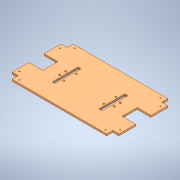
# Autodesk Inventor part: base
Saved by Autodesk Inventor 2020 (Build 240168000, 168)
## iProperties
Part Number: base
Material: Bois (cerisier)
Document SubType Name: Modeling
Designer: ElsaT
Density: 0.63 g/cm^3
Appearance: Cerisier - Faible lustre naturel
Author: ElsaT
Autodesk Inventor part; units mm, degrees
ref_plane "YZ Plane" through (0, 0, 0) normal (1, 0, 0) x (0, 1, 0)
ref_plane "XZ Plane" through (0, 0, 0) normal (0, 1, 0) x (-1, 0, 0)
ref_plane "XY Plane" through (0, 0, 0) normal (0, 0, 1) x (1, 0, 0)
sketch "Esquisse1" plane through (0, 0, 0) normal (0, 0, 1) x (1, 0, 0)
  line L0 (-155, -100) -> (155, -100)
  line L1 (175, -80) -> (175, 80)
  line L2 (155, 100) -> (-155, 100)
  line L3 (-175, 80) -> (-175, -80)
  line L4 (-175, -100) -> (175, 100) construction
  line L5 (175, -100) -> (-175, 100) construction
  line L6 (-155, 100) -> (-155, 80)
  line L7 (-155, 80) -> (-175, 80)
  line L8 (155, 100) -> (155, 80)
  line L9 (155, 80) -> (175, 80)
  line L10 (155, -100) -> (155, -80)
  line L11 (155, -80) -> (175, -80)
  line L12 (-155, -100) -> (-155, -80)
  line L13 (-155, -80) -> (-175, -80)
  circle A0 centre (-141, 90) radius 1.85
  circle A1 centre (-165, 66) radius 1.85
  circle A2 centre (-165, -66) radius 1.85
  circle A3 centre (-141, -90) radius 1.85
  circle A4 centre (141, 90) radius 1.85
  circle A5 centre (165, 66) radius 1.85
  circle A6 centre (165, -66) radius 1.85
  circle A7 centre (141, -90) radius 1.85
  point P0 (0, 0)
  dimension "d43" = 350
  dimension "d44" = 200
  dimension "d45" = 20
  dimension "d46" = 20
  dimension "d47" = 20
  dimension "d48" = 20
  dimension "d49" = 20
  dimension "d50" = 20
  dimension "d51" = 20
  dimension "d52" = 20
  dimension "d53" = 3.7
  dimension "d54" = 3.7
  dimension "d55" = 3.7
  dimension "d56" = 3.7
  dimension "d57" = 3.7
  dimension "d58" = 3.7
  dimension "d59" = 3.7
  dimension "d60" = 3.7
  dimension "d61" = 10
  dimension "d62" = 10
  dimension "d63" = 10
  dimension "d64" = 10
  dimension "d65" = 10
  dimension "d66" = 10
  dimension "d67" = 10
  dimension "d68" = 10
  dimension "d69" = 14
  dimension "d70" = 14
  dimension "d71" = 14
  dimension "d72" = 14
  dimension "d73" = 14
  dimension "d74" = 14
  dimension "d136" = 14
  dimension "d137" = 14
  constraints: 28 end point, 8 centre point, 7 horizontal, 2 midpoint, 2 parallel, 2 vertical, 1 perpendicular
  measures "d43" distance of L5.end L4.end
  measures "d44" distance of L4.end L5.start
  measures "d45" distance of L3.start L6.end
  measures "d46" distance of L2.end L6.end
  measures "d47" distance of L1.end L8.end
  measures "d48" distance of L2.start L8.end
  measures "d49" distance of L1.start L10.end
  measures "d50" distance of L0.end L10.end
  measures "d51" distance of L3.end L12.end
  measures "d52" distance of L0.start L12.end
  measures "d53" diameter of A0
  measures "d54" diameter of A1
  measures "d55" diameter of A2
  measures "d56" diameter of A3
  measures "d57" diameter of A4
  measures "d58" diameter of A5
  measures "d59" diameter of A6
  measures "d60" diameter of A7
  measures "d61" distance from line of L2 A0.centre
  measures "d62" distance from line of L3 A1.centre
  measures "d63" distance from line of L2 A4.centre
  measures "d64" distance from line of L1 A5.centre
  measures "d65" distance from line of L1 A6.centre
  measures "d66" distance from line of L0 A7.centre
  measures "d67" distance from line of L0 A3.centre
  measures "d68" distance from line of L3 A2.centre
  measures "d69" distance from line of L7 A1.centre
  measures "d70" distance from line of L6 A0.centre
  measures "d71" distance from line of L8 A4.centre
  measures "d72" distance from line of L9 A5.centre
  measures "d73" distance from line of L11 A6.centre
  measures "d74" distance from line of L10 A7.centre
  measures "d136" distance from line of L12 A3.centre
  measures "d137" distance from line of L13 A2.centre
extrude "Extrusion2" add sketch "Esquisse1" along normal blind 6
sketch "Esquisse3" plane through (0, 0, 6) normal (0, 0, 1) x (1, 0, 0)
  line L0 (175, -80) -> (175, 80) projected
  line L1 (175, -25) -> (175, 25)
  line L2 (175, 25) -> (130, 25)
  line L3 (130, 25) -> (130, -25)
  line L4 (130, -25) -> (175, -25)
  line L5 (155, 100) -> (-155, 100) projected
  line L6 (-175, -80) -> (-175, 80) projected
  line L7 (-175, -25) -> (-175, 25)
  line L8 (-175, 25) -> (-130, 25)
  line L9 (-130, 25) -> (-130, -25)
  line L10 (-130, -25) -> (-175, -25)
  point P0 (0, 0)
  dimension "d77" = 45
  dimension "d78" = 50
  dimension "d79" = 75
  dimension "d80" = 50
  dimension "d81" = 45
  constraints: 16 end point, 4 parallel, 4 point on line, 2 perpendicular
  measures "d77" distance of L2.end L1.end
  measures "d78" distance of L2.end L3.end
  measures "d79" distance between parallel lines of L5 L2
  measures "d80" distance of L7.start L7.end
  measures "d81" distance of L7.end L8.end
extrude "Extrusion3" cut sketch "Esquisse3" against normal blind 6
sketch "Esquisse4" plane through (0, 0, 6) normal (0, 0, 1) x (1, 0, 0)
  circle A0 centre (-89.5, 10) radius 3
  circle A1 centre (-89.5, -10) radius 3
  circle A2 centre (89.5, 10) radius 3
  circle A3 centre (89.5, -10) radius 3
  line L0 (-175, 80) -> (-175, 25) projected
  line L1 (-175, -25) -> (-175, -80) projected
  line L2 (175, 25) -> (175, 80) projected
  line L3 (175, -80) -> (175, -25) projected
  line L4 (155, 100) -> (-155, 100) projected
  line L5 (-155, -100) -> (155, -100) projected
  point P0 (0, 0)
  dimension "d84" = 6
  dimension "d85" = 6
  dimension "d86" = 6
  dimension "d87" = 6
  dimension "d88" = 85.5
  dimension "d89" = 85.5
  dimension "d90" = 85.5
  dimension "d91" = 85.5
  dimension "d92" = 90
  dimension "d93" = 90
  dimension "d94" = 90
  dimension "d95" = 90
  constraints: 4 centre point
  measures "d84" diameter of A0
  measures "d85" diameter of A1
  measures "d86" diameter of A2
  measures "d87" diameter of A3
  measures "d88" distance from line of L0 A0.centre
  measures "d89" distance from line of L1 A1.centre
  measures "d90" distance from line of L2 A2.centre
  measures "d91" distance from line of L3 A3.centre
  measures "d92" distance from line of A0.centre L4
  measures "d93" distance from line of L5 A1.centre
  measures "d94" distance from line of L4 A2.centre
  measures "d95" distance from line of L5 A3.centre
hole "Perçage2" at (-89.5, 10, 6) at (-89.5, -10, 6) at (89.5, 10, 6) at (89.5, -10, 6) direction (0, 0, -1) diameter 6 depth 8 tip angle 118
sketch "Esquisse5" plane through (0, 0, 6) normal (0, 0, 1) x (1, 0, 0)
  line L0 (-81.5, -42.5) -> (-71.5, -42.5)
  line L1 (-71.5, -42.5) -> (-71.5, 42.5)
  line L2 (-71.5, 42.5) -> (-81.5, 42.5)
  line L3 (-81.5, 42.5) -> (-81.5, -42.5)
  line L4 (-81.5, -42.5) -> (-71.5, 42.5) construction
  line L5 (-71.5, -42.5) -> (-81.5, 42.5) construction
  line L6 (-175, -25) -> (-175, -80) projected
  line L7 (71.5, -42.5) -> (81.5, -42.5)
  line L8 (81.5, -42.5) -> (81.5, 42.5)
  line L9 (81.5, 42.5) -> (71.5, 42.5)
  line L10 (71.5, 42.5) -> (71.5, -42.5)
  line L11 (71.5, -42.5) -> (81.5, 42.5) construction
  line L12 (81.5, -42.5) -> (71.5, 42.5) construction
  line L13 (130, 25) -> (130, -25) projected
  line L14 (175, -80) -> (175, -25) projected
  line L15 (-155, -100) -> (155, -100) projected
  point P0 (0, 0)
  point P1 (-76.5, 0)
  point P2 (76.5, 0)
  dimension "d103" = 10
  dimension "d104" = 85
  dimension "d107" = 10
  dimension "d108" = 85
  dimension "d111" = 100
  dimension "d112" = 100
  dimension "d134" = 93.5
  dimension "d135" = 93.5
  constraints: 24 end point, 4 midpoint, 4 parallel, 2 horizontal, 2 perpendicular
  measures "d103" distance of L2.end L1.end
  measures "d104" distance of L0.end L1.end
  measures "d107" distance of L9.end L8.end
  measures "d108" distance of L8.end L7.end
  measures "d111" distance from line of L15 point (-76.5, 0)
  measures "d112" distance from line of L15 point (76.5, 0)
  measures "d134" distance between parallel lines of L14 L8
  measures "d135" distance between parallel lines of L3 L6
extrude "Extrusion4" cut sketch "Esquisse5" against normal blind 6
sketch "Esquisse6" plane through (0, 0, 6) normal (0, 0, 1) x (1, 0, 0)
  circle A0 centre (-65, 20) radius 2.5
  circle A1 centre (-65, -20) radius 2.5
  circle A2 centre (65, 20) radius 2.5
  circle A3 centre (65, -20) radius 2.5
  line L0 (175, 25) -> (175, 80) projected
  line L1 (175, -80) -> (175, -25) projected
  line L2 (-175, 80) -> (-175, 25) projected
  line L3 (-175, -25) -> (-175, -80) projected
  line L4 (155, 100) -> (-155, 100) projected
  line L5 (-155, -100) -> (155, -100) projected
  point P0 (0, 0)
  dimension "d115" = 5
  dimension "d116" = 5
  dimension "d117" = 5
  dimension "d118" = 5
  dimension "d119" = 110
  dimension "d120" = 110
  dimension "d121" = 110
  dimension "d122" = 110
  dimension "d123" = 80
  dimension "d124" = 80
  dimension "d125" = 80
  dimension "d126" = 80
  constraints: 4 centre point
  measures "d115" diameter of A0
  measures "d116" diameter of A1
  measures "d117" diameter of A2
  measures "d118" diameter of A3
  measures "d119" distance from line of L0 A2.centre
  measures "d120" distance from line of L1 A3.centre
  measures "d121" distance from line of L2 A0.centre
  measures "d122" distance from line of L3 A1.centre
  measures "d123" distance from line of L4 A0.centre
  measures "d124" distance from line of L5 A1.centre
  measures "d125" distance from line of L5 A3.centre
  measures "d126" distance from line of L4 A2.centre
hole "Perçage3" at (-65, 20, 6) at (-65, -20, 6) at (65, 20, 6) at (65, -20, 6) direction (0, 0, -1) diameter 5 depth 8 tip angle 118
equation "\"d45\" = d51"
equation "\"d46\" = d51"
equation "\"d47\" = d52"
equation "\"d48\" = d51"
equation "\"d49\" = d52"
equation "\"d50\" = d52"
equation "\"d52\" = d51"
equation "\"d54\" = d53"
equation "\"d55\" = d53"
equation "\"d56\" = d53"
equation "\"d57\" = d53"
equation "\"d58\" = d53"
equation "\"d59\" = d53"
equation "\"d60\" = d53"
equation "\"d61\" = d62"
equation "\"d63\" = d62"
equation "\"d64\" = d62"
equation "\"d65\" = d62"
equation "\"d66\" = d62"
equation "\"d67\" = d62"
equation "\"d68\" = d62"
equation "\"d70\" = d69"
equation "\"d71\" = d69"
equation "\"d72\" = d69"
equation "\"d73\" = d69"
equation "\"d74\" = d69"
equation "\"d136\" = d74"
equation "\"d137\" = d69"
equation "\"d85\" = d84"
equation "\"d86\" = d84"
equation "\"d87\" = d84"
equation "\"d89\" = d88"
equation "\"d90\" = d88"
equation "\"d91\" = d88"
equation "\"d93\" = d92"
equation "\"d94\" = d92"
equation "\"d95\" = d93"
